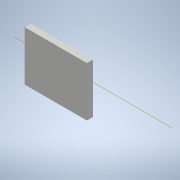
# Autodesk Inventor part: Крепление пружины
Saved by Autodesk Inventor 2020 (Build 240168000, 168)
## iProperties
Created: 2021-05-02
Part Number: Крепление пружины
Material: Типовые
Document SubType Name: Modeling
Designer: I_Love_U_Bogdan
Density: 1 g/cm^3
Appearance: По умолчанию
Author: I_Love_U_Bogdan
Autodesk Inventor part; units mm, degrees
ref_plane "YZ Plane" through (0, 0, 0) normal (1, 0, 0) x (0, 1, 0)
ref_plane "XZ Plane" through (0, 0, 0) normal (0, 1, 0) x (-1, 0, 0)
ref_plane "XY Plane" through (0, 0, 0) normal (0, 0, 1) x (1, 0, 0)
ref_plane "РабПлоскость1" through (0, 0, 0) normal (0, 0, 1) x (1, 0, 0)
sketch "Эскиз1" plane through (0, 0, 0) normal (0, 0, 1) x (1, 0, 0)
  line L0 (-10.8, -3.3341) -> (-10.8, 7.395) projected
  circle A0 centre (-13, 4.895) radius 1.5 projected
  line L1 (-11.5, 0.895) -> (-21.5, 0.895)
  line L2 (-21.5, 0.895) -> (-21.5, 8.895)
  line L3 (-21.5, 8.895) -> (-11.5, 8.895)
  line L4 (-11.5, 8.895) -> (-11.5, 0.895)
  point P0 (0, 0)
  dimension "d1" = 8
  dimension "d2" = 4
  dimension "d3" = 10
  constraints: 8 end point, 2 parallel, 1 horizontal, 1 perpendicular, 1 tangent
  measures "d1" distance of L1.end L2.end
  measures "d2" distance from line of L3 A0.centre
  measures "d3" distance of L1.start L1.end
extrude "Выдавливание1" add sketch "Эскиз1" along normal blind 0.4 contours A0 | L4 L1 L2 L3
sketch "Эскиз2" plane through (0, 0, 0.4) normal (0, 0, 1) x (1, 0, 0)
  line L0 (-11.5, 8.895) -> (-21.5, 8.895) projected
  line L1 (-21.5, 8.895) -> (-21.5, 0.895) projected
  line L2 (-21.5, 0.895) -> (-11.5, 0.895) projected
  line L3 (-11.5, 0.895) -> (-11.5, 8.895) projected
  line L4 (-11.5, 0.895) -> (-16.5, 0.895)
  line L5 (-16.5, 0.895) -> (-16.5, 8.895)
  line L6 (-16.5, 8.895) -> (-11.5, 8.895)
  line L7 (-11.5, 8.895) -> (-11.5, 0.895)
  point P0 (0, 0)
  point P1 (-16.5318, 8.895)
  dimension "d9" = 5
  constraints: 8 end point, 2 parallel, 1 horizontal, 1 midpoint, 1 perpendicular, 1 point on line
  measures "d9" distance of L5.end L6.end
extrude "Выдавливание2" add sketch "Эскиз2" along normal blind 0.6
equation "\"d2\" = 0.5 * d1"
